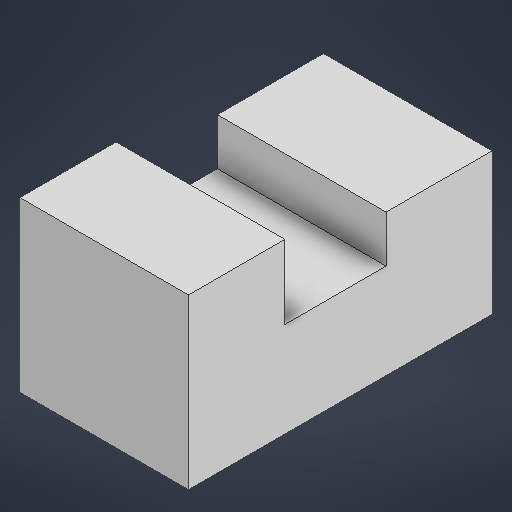
# Autodesk Inventor part: Peça2_aula
Saved by Autodesk Inventor 2026 (Build 300175000, 175)
## iProperties
Created: 2026-03-13
Part Number: Peça2_aula
Material: Genérico
Document SubType Name: Modeling
Designer: guisg
Density: 1 g/cm^3
Appearance: Padrão
Author: guisg
Autodesk Inventor part; units mm, degrees
ref_plane "YZ Plane" through (0, 0, 0) normal (1, 0, 0) x (0, 1, 0)
ref_plane "XZ Plane" through (0, 0, 0) normal (0, 1, 0) x (-1, 0, 0)
ref_plane "XY Plane" through (0, 0, 0) normal (0, 0, 1) x (1, 0, 0)
sketch "Esboço1" plane through (0, 0, 0) normal (1, 0, 0) x (0, 1, 0)
  line L0 (0, 0) -> (25, 0)
  line L1 (25, 0) -> (25, -45)
  line L2 (25, -45) -> (0, -45)
  line L3 (0, -45) -> (0, 0)
  dimension "d0" = 45
  dimension "d1" = 25
  constraints: 8 end point, 2 parallel, 1 horizontal, 1 perpendicular
  measures "d0" distance of L0.end L1.end
  measures "d1" distance of L1.end L2.end
extrude "Extrusão1" add sketch "Esboço1" along normal blind 25
sketch "Esboço4" plane through (0, 0, 0) normal (-1, 0, 0) x (0, 0, 1)
  line L0 (-29.275, 25) -> (-14.275, 25)
  line L1 (-14.275, 25) -> (-14.275, 14.0681)
  line L2 (-14.275, 14.0681) -> (-29.275, 14.0681)
  line L3 (-29.275, 14.0681) -> (-29.275, 25)
  line L4 (0, 0) -> (-45, 0) projected
  dimension "d8" = 25
  dimension "d9" = 15
  constraints: 8 end point, 2 parallel, 1 horizontal, 1 perpendicular
  measures "d8" distance between parallel lines of L4 L0
  measures "d9" distance between parallel lines of L3 L1
extrude "Extrusão3" cut sketch "Esboço4" against normal through all
sketch "Esboço6" plane through (0, 0, 0) normal (-1, 0, 0) x (0, 0, 1)
  line L0 (-45, 25) -> (-29.275, 25) projected
  line L1 (-29.275, 14.0681) -> (-29.275, 25) projected
  line L2 (-45, 25) -> (-29.275, 25)
  line L3 (-29.275, 25) -> (-29.275, 21)
  line L4 (-29.275, 21) -> (-45, 21)
  line L5 (-45, 21) -> (-45, 25)
  point P0 (0, 0)
  point P1 (-37.1375, 21)
  dimension "d12" = 4
  dimension "d13" = 15.725
  constraints: 8 end point, 2 parallel, 1 horizontal, 1 midpoint, 1 perpendicular, 1 point on line
  measures "d12" distance from line of point (-37.137, 21) L0
  measures "d13" distance between parallel lines of L1 L5
extrude "Extrusão4" cut sketch "Esboço6" against normal through all
